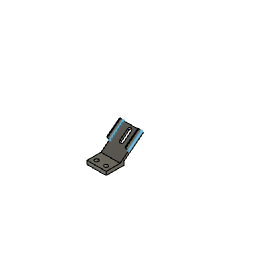
sensor_holder (Autodesk Fusion 360 design; units mm, degrees)
Autodesk Fusion 360 part; units mm, degrees
sketch "Sketch1" plane through (0, 0, 0) normal (0, 0, 1) x (-1, 0, 0)
  line L0 (25.425, -51.5372) -> (25.425, -27.0727)
  arc A0 (28.575, -27.0727) -> (25.425, -27.0727) centre (27, -27.0727) ccw
  line L1 (28.575, -27.0727) -> (28.575, -51.5372)
  arc A1 (25.425, -51.5372) -> (28.575, -51.5372) centre (27, -51.5372) ccw
  line L2 (17.425, -51.5372) -> (17.425, -27.0727)
  arc A2 (20.575, -27.0727) -> (17.425, -27.0727) centre (19, -27.0727) ccw
  line L3 (20.575, -27.0727) -> (20.575, -51.5372)
  arc A3 (17.425, -51.5372) -> (20.575, -51.5372) centre (19, -51.5372) ccw
  circle A4 centre (12.9152, -52.7872) radius 1.75
  circle A5 centre (12.9152, -25.8227) radius 1.75
  line L4 (30.1652, -22.0727) -> (9.1652, -22.0727)
  line L5 (9.1652, -22.0727) -> (9.1652, -29.5727)
  line L6 (9.1652, -29.5727) -> (9.1652, -49.0372)
  line L7 (9.1652, -49.0372) -> (9.1652, -56.5372)
  line L8 (9.1652, -56.5372) -> (30.1652, -56.5372)
  line L9 (30.1652, -56.5372) -> (30.1652, -22.0727)
  circle A6 centre (27, -27.0727) radius 1.575
  circle A7 centre (19, -27.0727) radius 1.575
  line L10 (19, -27.0727) -> (27, -27.0727) construction
  line L11 (23, -27.0727) -> (23, -22.0727) construction
  line L12 (23, -23.0727) -> (15, -23.0727)
  line L13 (15, -23.0727) -> (15, -38.0727)
  line L14 (15, -38.0727) -> (23, -38.0727)
  line L15 (23, -27.0727) -> (23, -38.0727) construction
  line L16 (31, -38.0727) -> (23, -38.0727)
  line L17 (31, -23.0727) -> (31, -38.0727)
  line L18 (23, -23.0727) -> (31, -23.0727)
  dimension "d313" = 8
  dimension "d314" = 15
  dimension "d315" = 4
  constraint concentric A0 A6
  constraint concentric A2 A7
  constraint coincident A2.centre A7.centre
  constraint coincident A0.centre A6.centre
  constraint midpoint L10 L11.start
  constraint perpendicular L10 L11
  constraint coincident L4 L11.end
  constraint coincident L11 L12.start
  constraint perpendicular L11 L12
  constraint perpendicular L3 L14
  constraint perpendicular L14 L15
  constraint coincident L14.end L15.end
  constraint parallel L3 L13
  constraint symmetric L12.start L15 L18.start
  constraint symmetric L12.end L15 L17.start
  constraint symmetric L13.end L15 L16.start
  constraint symmetric L14.end L15 L16.end
  constraint equal A0 A6
  constraint equal A2 A7
  measures "d313" distance of L12.start L12.end
  measures "d314" distance of L12.end L13.end
  measures "d315" distance of A2.centre L12
extrude "Extrude1" add sketch "Sketch1" along normal blind 3 contours L0 A0 L1 L2 A2 L3 L9 A6 A7 L12 L13 L14 L16 L18 | L0 L1 A6 L16 | L9 L16 L17 L18 | L2 L3 A7 L14
sketch "Sketch2" plane through (-15, 0, 0) normal (1, 0, 0) x (0, 1, 0)
  line L0 (23.0727, 0) -> (38.0727, 0)
  line L1 (38.0727, 0) -> (38.0727, 3)
  line L2 (38.0727, 3) -> (23.0727, 3)
  line L3 (23.0727, 3) -> (23.0727, 0)
sketch "Sketch3" plane through (-31, 0, 0) normal (-1, 0, 0) x (0, -1, 0)
  line L0 (-38.0727, 0) -> (-23.0727, 0)
  line L1 (-23.0727, 0) -> (-23.0727, 3)
  line L2 (-23.0727, 3) -> (-38.0727, 3)
  line L3 (-38.0727, 3) -> (-38.0727, 0)
  line L4 (-34.8242, 3) -> (-52.9484, 17.1602)
  line L5 (-52.9484, 17.1602) -> (-54.1797, 15.5842)
  line L6 (-54.1797, 15.5842) -> (-38.0727, 3)
  line L7 (-38.0727, 3) -> (-34.8242, 3)
  dimension "d318" = 38
  dimension "d319" = 23
  dimension "d320" = 2
  constraint perpendicular L4 L5
  constraint perpendicular L5 L6
  constraint coincident L2 L4.start
  constraint coincident L2.end L3.start
  measures "d318" angle of L2 L4
  measures "d319" distance of L4.start L4.end
  measures "d320" distance of L4 L6
extrude "Extrude2" add sketch "Sketch3" against normal up to surface (16 mm away) contours L2 L4 L5 L6 L7
sketch "Sketch4" plane through (0, 11.7443, -15.032) normal (0, -0.615661, 0.788011) x (1, 0, 0)
  line L0 (-15, 29.2888) -> (-15, 52.2888)
  line L1 (-15, 52.2888) -> (-31, 52.2888)
  line L2 (-31, 52.2888) -> (-31, 29.2888)
  line L3 (-31, 29.2888) -> (-15, 29.2888)
  line L4 (-23, 52.2888) -> (-23, 29.2888) construction
  circle A0 centre (-23, 49.2888) radius 1.575
  circle A1 centre (-23, 41.2888) radius 1.575
  line L5 (-21.425, 49.2888) -> (-21.425, 41.2888)
  line L6 (-24.575, 49.2888) -> (-24.575, 41.2888)
  dimension "d323" = 3.15
  dimension "d324" = 8
  dimension "d325" = 3
  constraint midpoint L1 L4.start
  constraint midpoint L3 L4.end
  constraint coincident L4 A0.centre
  constraint coincident L4 A1.centre
  constraint equal A0 A1
  constraint coincident A0 L5.start
  constraint coincident A1 L5.end
  constraint tangent A1 L5
  constraint coincident A0 L6.start
  constraint coincident A1 L6.end
  constraint parallel L4 L6
  constraint tangent A0 L5
  constraint tangent A0 L6
  measures "d323" diameter of A0
  measures "d324" distance of A0.centre A1.centre
  measures "d325" distance of L1 A0.centre
extrude "Extrude3" cut sketch "Sketch4" against normal up to surface (2 mm away) contours A0 | A0 A1 L5 L6 | A1
sketch "sketch 1086" plane through (0, 7.3976, -18.428) normal (0, -0.615661, 0.788011) x (1, 0, 0)
  line L0 (-15.7, 43.8049) -> (-15, 43.8049)
  line L1 (-15, 43.8049) -> (-15, 57.8049)
  line L2 (-15, 43.8049) -> (-15, 57.8049)
  line L3 (-15, 57.8049) -> (-15.7, 57.8049)
  line L4 (-15.7, 57.8049) -> (-15.7, 43.8049)
  line L5 (-30.3, 43.8049) -> (-31, 43.8049)
  line L6 (-30.3, 57.8049) -> (-30.3, 43.8049)
  line L7 (-31, 57.8049) -> (-30.3, 57.8049)
  line L8 (-31, 57.8049) -> (-30.3, 57.8049)
  line L9 (-31, 43.8049) -> (-31, 57.8049)
  line L10 (-31, 43.8049) -> (-31, 57.8049)
extrude "Extrude4" add sketch "sketch 1086" along normal blind 4
